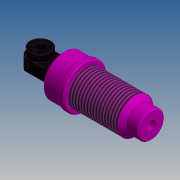
# Autodesk Inventor part: Corps
Saved by Autodesk Inventor 2021.3 (Build 253353000, 353)
## iProperties
Created: 2023-04-12
Part Number: Corps
Material: Aluminum 6061
Document SubType Name: Modeling
Designer: cedric.clivaz
Density: 2.7 g/cm^3
Appearance: Magenta
Author: cedric.clivaz
Autodesk Inventor part; units mm, degrees
ref_plane "YZ Plane" through (0, 0, 0) normal (1, 0, 0) x (0, 1, 0)
ref_plane "XZ Plane" through (0, 0, 0) normal (0, 1, 0) x (-1, 0, 0)
ref_plane "XY Plane" through (0, 0, 0) normal (0, 0, 1) x (1, 0, 0)
sketch "Sketch2" plane through (0, 0, 0) normal (0, 0, 1) x (1, 0, 0)
  line L0 (-6.1, 0) -> (36.6, 0) construction
  line L1 (0, -1.48) -> (0, 8.88) construction
  line L2 (0, 0) -> (0, 7)
  line L3 (0, 7) -> (6, 7)
  line L4 (6, 7) -> (6, 7.4)
  line L5 (6, 7.4) -> (8, 7.4)
  line L6 (8, 7.4) -> (8, 6)
  line L7 (8, 6) -> (26.5, 6)
  line L8 (26.5, 6) -> (26.5, 4.5)
  line L9 (26.5, 4.5) -> (30.5, 4.5)
  line L10 (30.5, 4.5) -> (30.5, 0)
  line L11 (0, 0) -> (30.5, 0)
  dimension "d0" = 14
  dimension "d1" = 30.5
  dimension "d2" = 8
  dimension "d3" = 14.8
  dimension "d4" = 9
  dimension "d5" = 4
  dimension "d6" = 12
  dimension "d7" = 6
  constraints: 20 end point, 9 perpendicular, 2 collinear, 2 point on line
  measures "d0" diameter of L3 L0
  measures "d1" distance between parallel lines of L10 L2
  measures "d2" distance between parallel lines of L2 L6
  measures "d3" diameter of L5 L0
  measures "d4" diameter of L9 L0
  measures "d5" distance between parallel lines of L8 L10
  measures "d6" diameter of L7 L0
  measures "d7" distance of L2.end L3.end
revolve "Revolution1" add sketch "Sketch2" angle 360 about axis through (-10, 0, 0) along (1, 0, 0)
thread "Thread1" size "M12x1" class "6g" standard "ISO Metric profile" length 110
chamfer "Chamfer1" distance 1.5 angle 45 1 edges at (26.5, -6, 0)
chamfer "Chamfer2" distance 0.4 angle 45 3 edges at (6, -7.4, 0) (8, -7.4, 0) (30.5, -4.5, 0)
chamfer "Chamfer3" distance 1 angle 45 1 edges at (0, -7, 0)
sketch "Sketch3" plane through (0, 0, 0) normal (-1, 0, 0) x (0, 0, 1)
  circle A0 centre (0, 0) radius 4
  dimension "d20" = 8
  constraints: 1 centre point, 1 coincident
  measures "d20" diameter of A0
extrude "Extrusion1" add sketch "Sketch3" along normal blind 11.3
sketch "Sketch4" plane through (-11.3, 0, 0) normal (-1, 0, 0) x (0, 0, 1)
  line L0 (0, -10.36) -> (0, 10.36) construction
  circle A0 centre (0, 0) radius 4 construction
  circle A1 centre (0, 0) radius 4
  line L1 (-2, -3.4641) -> (-2, 3.4641)
  line L2 (2, 3.4641) -> (2, -3.4641)
  dimension "d23" = 4
  constraints: 4 end point, 4 point on circle, 1 centre point, 1 coincident, 1 concentric, 1 parallel, 1 vertical, 1 other
  measures "d23" distance between parallel lines of L1 L2
extrude "Extrusion2" cut sketch "Sketch4" against normal blind 10 contours A1 L2 | L1 A1
sketch "Sketch5" plane through (-11.3, -3.4641, 2) normal (0, 0, 1) x (1, 0, 0)
  line L0 (-8.36, 3.4641) -> (50.16, 3.4641) construction
  circle A0 centre (4, 3.4641) radius 4
  line L1 (0, 0) -> (0, 6.9282) construction
  line L2 (10, 0) -> (0, 0) construction
  line L3 (10, 0) -> (10, 6.9282) construction
  line L4 (0, 6.9282) -> (10, 6.9282) construction
  line L5 (0, 0) -> (0, 6.9282) construction
  line L6 (11.3, 7.4641) -> (0, 7.4641) construction
  line L7 (11.3, -0.5359) -> (0, -0.5359) construction
  line L8 (4, -0.5359) -> (0, -0.5359)
  line L9 (0, -0.5359) -> (0, 7.4641)
  line L10 (0, 7.4641) -> (4, 7.4641)
  point P0 (11.3, 3.4641)
  point P1 (0, 3.4641)
  dimension "d26" = 8
  constraints: 6 end point, 3 point on line, 2 collinear, 2 point on circle, 1 centre point, 1 tangent
  measures "d26" diameter of A0
extrude "Extrusion3" cut sketch "Sketch5" against normal through all contours A0 L9 L10 | L8 L9 A0
sketch "Sketch6" plane through (-1.3, -3.4641, 2) normal (0, 0, 1) x (1, 0, 0)
  arc A0 (-8, 6.9282) -> (-8, 0) centre (-6, 3.4641) ccw construction
  circle A1 centre (-6, 3.4641) radius 1.5
  point P0 (1.3, 3.4641)
  dimension "d29" = 3
  constraints: 1 centre point, 1 coincident
  measures "d29" diameter of A1
extrude "Extrusion4" cut sketch "Sketch6" against normal through all
sketch "Sketch7" plane through (-1.3, -3.4641, 2) normal (0, 0, 1) x (1, 0, 0)
  circle A0 centre (-6, 3.4641) radius 1.5 construction
  circle A1 centre (-6, 3.4641) radius 1.5
  circle A2 centre (-6, 3.4641) radius 3.5
  point P0 (1.3, 3.4641)
  dimension "d32" = 7
  constraints: 2 centre point, 2 coincident, 1 concentric
  measures "d32" diameter of A2
extrude "Extrusion5" add sketch "Sketch7" along normal blind 2.3
sketch "Sketch8" plane through (30.5, 0, 0) normal (1, 0, 0) x (0, 0, -1)
  circle A0 centre (0, 0) radius 1.5
  dimension "d35" = 3
  constraints: 1 centre point, 1 coincident
  measures "d35" diameter of A0
extrude "Extrusion6" cut sketch "Sketch8" against normal blind 20
body "Solid1"
